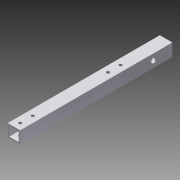
# Autodesk Inventor part: 1x1 lengthwise
Saved by Autodesk Inventor 2015 SP1 (Build 190203100, 203)
## iProperties
Created: 2015-01-27
Part Number: 1x1 lengthwise
Material: Aluminum 6061
Document SubType Name: Modeling
Designer: Admin
Density: 2.7 g/cm^3
Appearance: Aluminum - Flat
Author: Admin
Autodesk Inventor part; units mm, degrees
ref_plane "YZ Plane" through (0, 0, 0) normal (1, 0, 0) x (0, 1, 0)
ref_plane "XZ Plane" through (0, 0, 0) normal (0, 1, 0) x (-1, 0, 0)
ref_plane "XY Plane" through (0, 0, 0) normal (0, 0, 1) x (1, 0, 0)
sketch "Sketch1" plane through (0, 0, 0) normal (0, 0, 1) x (1, 0, 0)
  line L0 (0, 0) -> (25.4, 0)
  line L1 (25.4, 0) -> (25.4, 25.4)
  line L2 (25.4, 25.4) -> (0, 25.4)
  line L3 (0, 25.4) -> (0, 0)
  line L4 (3.175, 3.175) -> (22.225, 3.175)
  line L5 (22.225, 3.175) -> (22.225, 22.225)
  line L6 (22.225, 22.225) -> (3.175, 22.225)
  line L7 (3.175, 22.225) -> (3.175, 3.175)
  dimension "d0" = 25.4
  dimension "d1" = 25.4
  dimension "d2" = 19.05
  dimension "d3" = 19.05
  dimension "d4" = 3.175
  dimension "d5" = 3.175
  constraints: 16 end point, 4 parallel, 2 horizontal, 2 perpendicular
  measures "d0" distance of L2.end L1.end
  measures "d1" distance of L1.end L0.end
  measures "d2" distance of L6.end L5.end
  measures "d3" distance of L5.end L4.end
  measures "d4" distance between parallel lines of L0 L4
  measures "d5" distance between parallel lines of L7 L3
extrude "Extrusion1" add sketch "Sketch1" along normal blind 307.975
sketch "Sketch2" plane through (0, 25.4, 0) normal (0, 1, 0) x (1, 0, 0)
  line L0 (25.4, -307.975) -> (0, -307.975) projected
  line L1 (25.4, 0) -> (25.4, -307.975) projected
  point P0 (12.7, -295.275)
  point P1 (12.7, -269.875)
  point P2 (12.7, -117.475)
  point P3 (12.7, -92.075)
  dimension "d8" = 12.7
  dimension "d9" = 12.7
  dimension "d11" = 12.7
  dimension "d16" = 12.7
  dimension "d17" = 12.7
  dimension "d34" = 152.4
  dimension "d35" = 25.4
  dimension "d36" = 25.4
  measures "d8" distance from line of L0 point (12.7, -295.275)
  measures "d9" distance from line of L1 point (12.7, -295.275)
  measures "d11" distance from line of L1 point (12.7, -269.875)
  measures "d16" distance from line of L1 point (12.7, -92.075)
  measures "d17" distance from line of L1 point (12.7, -117.475)
  measures "d34" distance of point (12.7, -269.875) point (12.7, -117.475)
  measures "d35" distance of point (12.7, -92.075) point (12.7, -117.475)
  measures "d36" distance of point (12.7, -295.275) point (12.7, -269.875)
hole "Hole1" at (12.7, 25.4, 295.275) at (12.7, 25.4, 269.875) at (12.7, 25.4, 117.475) at (12.7, 25.4, 92.075) direction (0, -1, 0) diameter 6.35 end through all
sketch "Sketch3" plane through (25.4, 0, 0) normal (1, 0, 0) x (0, 0, -1)
  line L0 (0, 0) -> (0, 25.4) projected
  line L1 (0, 0) -> (-307.975, 0) projected
  point P0 (-38.1, 12.7)
  dimension "d25" = 38.1
  dimension "d26" = 12.7
  measures "d25" distance from line of L0 point (-38.1, 12.7)
  measures "d26" distance from line of L1 point (-38.1, 12.7)
hole "Hole2" at (25.4, 12.7, 38.1) direction (-1, 0, 0) diameter 9.525 end through all
sketch "Sketch4" plane through (0, 0, 0) normal (-1, 0, 0) x (0, 0, 1)
  circle A0 centre (38.1, 12.7) radius 4.7625 projected
  circle A1 centre (38.1, 12.7) radius 6.35
  dimension "d37" = 12.7
  constraints: 1 centre point, 1 coincident
  measures "d37" diameter of A1
extrude "Extrusion2" cut sketch "Sketch4" against normal blind 12.7
body "Solid1"
